Autodesk Fusion 360 part; units mm, degrees
(part 7 of 7)
  spline S1999 degree 3 poles (64.4203, 41.5434) (64.0986, 41.5432) (63.8013, 41.7148) (63.6405, 41.9935) knots 0 0 0 0 1 1 1 1
  spline S2000 degree 3 poles (60.9466, 43.3939) (61.0983, 43.3207) (61.2414, 43.2308) (61.373, 43.1257) knots 0 0 0 0 1 1 1 1
  spline S2001 degree 3 poles (61.9187, 40.2416) (61.7213, 39.8998) (61.4373, 39.6159) (61.0955, 39.4184) knots 0 0 0 0 1 1 1 1
  spline S2002 degree 3 poles (59.9705, 43.6166) (60.1388, 43.6166) (60.3066, 43.5977) (60.4707, 43.5603) knots 0 0 0 0 1 1 1 1
  line L833 (55.8472, 45.7565) -> (55.8472, 45.7565)
  spline S2003 degree 3 poles (59.9705, 39.1166) (59.5755, 39.1167) (59.1875, 39.2208) (58.8455, 39.4184) knots 0 0 0 0 1 1 1 1
  spline S2004 degree 3 poles (63.6405, 42.8937) (63.8013, 43.1723) (64.0986, 43.3439) (64.4203, 43.3438) knots 0 0 0 0 1 1 1 1
  spline S2005 degree 3 poles (61.0955, 39.4184) (60.7535, 39.2208) (60.3655, 39.1167) (59.9705, 39.1166) knots 0 0 0 0 1 1 1 1
  spline S2006 degree 3 poles (50.3545, 46.2686) (49.8082, 46.2688) (49.2842, 46.0518) (48.8978, 45.6656) knots 0 0 0 0 1 1 1 1
  spline S2007 degree 3 poles (42.1917, 76.9836) (42.4279, 76.7471) (42.7484, 76.6142) (43.0826, 76.6141) knots 0 0 0 0 1 1 1 1
  spline S2008 degree 3 poles (58.0218, 40.2416) (57.8243, 40.5837) (57.7204, 40.9717) (57.7205, 41.3666) knots 0 0 0 0 1 1 1 1
  spline S2009 degree 3 poles (58.8455, 43.3153) (59.1875, 43.5128) (59.5755, 43.6167) (59.9705, 43.6166) knots 0 0 0 0 1 1 1 1
  spline S2010 degree 3 poles (58.0218, 42.4916) (58.2193, 42.8337) (58.5034, 43.1178) (58.8455, 43.3153) knots 0 0 0 0 1 1 1 1
  line L834 (59.9705, 43.6166) -> (59.9705, 43.6166)
  spline S2011 degree 3 poles (61.9972, 42.3433) (62.0704, 42.1914) (62.1262, 42.0317) (62.1636, 41.8674) knots 0 0 0 0 1 1 1 1
  line L835 (55.8472, 45.7565) -> (55.8472, 45.7565)
  spline S2012 degree 3 poles (83.1654, 44.538) (83.291, 44.4972) (83.4095, 44.4368) (83.5163, 44.3592) knots 0 0 0 0 1 1 1 1
  spline S2013 degree 3 poles (54.9563, 45.3876) (55.1926, 45.6238) (55.5131, 45.7565) (55.8472, 45.7565) knots 0 0 0 0 1 1 1 1
  line L836 (64.4203, 43.3438) -> (64.4203, 43.3438)
  spline S2014 degree 3 poles (61.373, 43.1257) (61.5048, 43.0207) (61.6244, 42.9013) (61.7295, 42.7696) knots 0 0 0 0 1 1 1 1
  spline S2015 degree 3 poles (60.4707, 43.5603) (60.6351, 43.5228) (60.7947, 43.467) (60.9466, 43.3939) knots 0 0 0 0 1 1 1 1
  spline S2016 degree 3 poles (14.7696, 50.8405) (14.7523, 50.8869) (14.7334, 50.9328) (14.7128, 50.9779) knots 0 0 0 0 1 1 1 1
  spline S2017 degree 3 poles (56.7381, 43.6058) (56.5018, 43.3695) (56.1814, 43.2368) (55.8472, 43.2368) knots 0 0 0 0 1 1 1 1
  spline S2018 degree 3 poles (61.7295, 42.7696) (61.8344, 42.638) (61.9242, 42.495) (61.9972, 42.3433) knots 0 0 0 0 1 1 1 1
  spline S2019 degree 3 poles (55.8472, 43.2368) (55.5131, 43.2368) (55.1926, 43.3695) (54.9563, 43.6058) knots 0 0 0 0 1 1 1 1
  spline S2020 degree 3 poles (58.8455, 39.4184) (58.5034, 39.6158) (58.2193, 39.8997) (58.0218, 40.2416) knots 0 0 0 0 1 1 1 1
  spline S2021 degree 3 poles (57.7205, 41.3666) (57.7204, 41.7616) (57.8243, 42.1496) (58.0218, 42.4916) knots 0 0 0 0 1 1 1 1
  spline S2022 degree 3 poles (83.5163, 44.3592) (83.6234, 44.2814) (83.7176, 44.1872) (83.7954, 44.0802) knots 0 0 0 0 1 1 1 1
  spline S2023 degree 3 poles (42.1917, 78.7654) (41.9555, 78.5291) (41.8227, 78.2086) (41.8228, 77.8745) knots 0 0 0 0 1 1 1 1
  spline S2024 degree 3 poles (57.1071, 44.4967) (57.1071, 44.1625) (56.9744, 43.8421) (56.7381, 43.6058) knots 0 0 0 0 1 1 1 1
  spline S2025 degree 3 poles (54.9563, 45.3876) (54.7199, 45.1514) (54.587, 44.8309) (54.5868, 44.4967) knots 0 0 0 0 1 1 1 1
  spline S2026 degree 3 poles (57.0456, 44.8858) (57.0046, 45.0116) (56.9441, 45.1302) (56.8663, 45.2372) knots 0 0 0 0 1 1 1 1
  spline S2027 degree 3 poles (70.6081, 44.2538) (70.7821, 44.3003) (70.9492, 44.3695) (71.1052, 44.4595) knots 0 0 0 0 1 1 1 1
  spline S2028 degree 3 poles (54.9563, 43.6058) (55.1926, 43.3695) (55.5131, 43.2368) (55.8472, 43.2368) knots 0 0 0 0 1 1 1 1
  line L837 (72.069, 46.7436) -> (71.5853, 46.7436)
  spline S2029 degree 3 poles (71.5093, 39.8938) (71.3486, 39.6154) (71.0515, 39.4438) (70.73, 39.4437) knots 0 0 0 0 1 1 1 1
  line L838 (71.5853, 46.7436) -> (71.5853, 47.6303)
  spline S2030 degree 3 poles (68.6407, 39.8938) (68.4801, 40.1722) (68.4801, 40.5151) (68.6407, 40.7935) knots 0 0 0 0 1 1 1 1
  spline S2031 degree 3 poles (64.4203, 43.3438) (64.0986, 43.3439) (63.8013, 43.1723) (63.6405, 42.8937) knots 0 0 0 0 1 1 1 1
  line L839 (69.42, 41.2436) -> (69.42, 41.2436)
  spline S2032 degree 3 poles (71.1052, 48.0277) (70.9492, 48.1177) (70.7821, 48.1869) (70.6081, 48.2334) knots 0 0 0 0 1 1 1 1
  spline S2033 degree 3 poles (71.5315, 44.7871) (71.6589, 44.9143) (71.769, 45.0576) (71.8592, 45.2134) knots 0 0 0 0 1 1 1 1
  spline S2034 degree 3 poles (63.6839, 45.3524) (63.9202, 45.1162) (64.2407, 44.9834) (64.5748, 44.9835) knots 0 0 0 0 1 1 1 1
  spline S2035 degree 3 poles (71.8592, 45.2134) (71.9492, 45.3694) (72.0183, 45.5366) (72.0648, 45.7105) knots 0 0 0 0 1 1 1 1
  spline S2036 degree 3 poles (65.5944, 46.9844) (65.5168, 47.0912) (65.4228, 47.1852) (65.3159, 47.2629) knots 0 0 0 0 1 1 1 1
  spline S2037 degree 3 poles (57.1071, 44.4967) (57.1071, 44.6288) (57.0864, 44.7601) (57.0456, 44.8858) knots 0 0 0 0 1 1 1 1
  spline S2038 degree 3 poles (70.0753, 44.1835) (70.2552, 44.1836) (70.4343, 44.2072) (70.6081, 44.2538) knots 0 0 0 0 1 1 1 1
  spline S2039 degree 3 poles (56.8663, 45.2372) (56.7886, 45.3441) (56.6946, 45.4381) (56.5877, 45.5157) knots 0 0 0 0 1 1 1 1
  spline S2040 degree 3 poles (64.5748, 44.9835) (64.9092, 44.9833) (65.2298, 45.116) (65.4663, 45.3524) knots 0 0 0 0 1 1 1 1
  spline S2041 degree 3 poles (81.5159, 43.3396) (81.5159, 43.6738) (81.6486, 43.9942) (81.8849, 44.2305) knots 0 0 0 0 1 1 1 1
  spline S2042 degree 3 poles (72.0648, 45.7105) (72.1115, 45.8845) (72.1351, 46.0638) (72.1351, 46.2438) knots 0 0 0 0 1 1 1 1
  spline S2043 degree 3 poles (72.1351, 46.2438) (72.1336, 46.4125) (72.1114, 46.5803) (72.069, 46.7436) knots 0 0 0 0 1 1 1 1
  spline S2044 degree 3 poles (63.6839, 47.1347) (63.4477, 46.8984) (63.315, 46.578) (63.315, 46.2438) knots 0 0 0 0 1 1 1 1
  spline S2045 degree 3 poles (65.4663, 45.3524) (65.7026, 45.5888) (65.8354, 45.9095) (65.8352, 46.2438) knots 0 0 0 0 1 1 1 1
  spline S2046 degree 3 poles (71.5853, 47.6303) (71.5679, 47.654) (71.5499, 47.6772) (71.5315, 47.7001) knots 0 0 0 0 1 1 1 1
  spline S2047 degree 3 poles (84.0357, 43.3396) (84.0357, 43.0055) (83.903, 42.685) (83.6667, 42.4487) knots 0 0 0 0 1 1 1 1
  spline S2048 degree 3 poles (83.6667, 42.4487) (83.4304, 42.2125) (83.1099, 42.0798) (82.7758, 42.0798) knots 0 0 0 0 1 1 1 1
  spline S2049 degree 3 poles (81.8849, 42.4487) (81.6486, 42.685) (81.5159, 43.0055) (81.5159, 43.3396) knots 0 0 0 0 1 1 1 1
  spline S2050 degree 3 poles (56.7381, 43.6058) (56.9744, 43.8421) (57.1071, 44.1625) (57.1071, 44.4967) knots 0 0 0 0 1 1 1 1
  spline S2051 degree 3 poles (63.6405, 42.8937) (63.4797, 42.6151) (63.4797, 42.272) (63.6405, 41.9935) knots 0 0 0 0 1 1 1 1
  spline S2052 degree 3 poles (55.8472, 45.7565) (55.5131, 45.7565) (55.1926, 45.6238) (54.9563, 45.3876) knots 0 0 0 0 1 1 1 1
  spline S2053 degree 3 poles (56.5877, 45.5157) (56.4808, 45.5936) (56.3622, 45.6541) (56.2363, 45.695) knots 0 0 0 0 1 1 1 1
  spline S2054 degree 3 poles (55.8472, 43.2368) (56.1814, 43.2368) (56.5018, 43.3695) (56.7381, 43.6058) knots 0 0 0 0 1 1 1 1
  line L840 (70.73, 39.4437) -> (69.42, 39.4437)
  spline S2055 degree 3 poles (71.5315, 47.7001) (71.4043, 47.8274) (71.261, 47.9376) (71.1052, 48.0277) knots 0 0 0 0 1 1 1 1
  spline S2056 degree 3 poles (68.6407, 40.7935) (68.8015, 41.072) (69.0985, 41.2436) (69.42, 41.2436) knots 0 0 0 0 1 1 1 1
  spline S2057 degree 3 poles (68.6185, 44.7871) (69.0048, 44.4006) (69.5289, 44.1835) (70.0753, 44.1835) knots 0 0 0 0 1 1 1 1
  spline S2058 degree 3 poles (63.6405, 41.9935) (63.8013, 41.7148) (64.0986, 41.5432) (64.4203, 41.5434) knots 0 0 0 0 1 1 1 1
  line L841 (64.4203, 41.5434) -> (65.7303, 41.5434)
  spline S2059 degree 3 poles (66.5096, 41.9935) (66.6705, 42.272) (66.6705, 42.6151) (66.5096, 42.8937) knots 0 0 0 0 1 1 1 1
  spline S2060 degree 3 poles (69.42, 39.4437) (69.0985, 39.4438) (68.8015, 39.6154) (68.6407, 39.8938) knots 0 0 0 0 1 1 1 1
  spline S2061 degree 3 poles (70.0753, 48.3037) (69.5289, 48.3036) (69.0048, 48.0865) (68.6185, 47.7001) knots 0 0 0 0 1 1 1 1
  spline S2062 degree 3 poles (68.0149, 46.2438) (68.015, 45.6974) (68.2321, 45.1734) (68.6185, 44.7871) knots 0 0 0 0 1 1 1 1
  line L842 (64.5748, 47.5037) -> (64.5748, 47.5037)
  spline S2063 degree 3 poles (66.5096, 42.8937) (66.3489, 43.1721) (66.0518, 43.3437) (65.7303, 43.3438) knots 0 0 0 0 1 1 1 1
  line L843 (65.7303, 43.3438) -> (64.4203, 43.3438)
  spline S2064 degree 3 poles (64.5748, 47.5037) (64.2407, 47.5037) (63.9202, 47.371) (63.6839, 47.1347) knots 0 0 0 0 1 1 1 1
  spline S2065 degree 3 poles (54.5868, 44.4967) (54.587, 44.1624) (54.7199, 43.842) (54.9563, 43.6058) knots 0 0 0 0 1 1 1 1
  spline S2066 degree 3 poles (126.6656, 70.8227) (126.2016, 70.8226) (125.7566, 70.6382) (125.4285, 70.3101) knots 0 0 0 0 1 1 1 1
  spline S2067 degree 3 poles (125.4285, 70.3101) (125.1003, 69.982) (124.9159, 69.537) (124.9159, 69.0729) knots 0 0 0 0 1 1 1 1
  spline S2068 degree 3 poles (64.9645, 47.4417) (64.8387, 47.4827) (64.7072, 47.5036) (64.5748, 47.5037) knots 0 0 0 0 1 1 1 1
  spline S2069 degree 3 poles (126.6656, 67.3227) (127.1298, 67.3226) (127.575, 67.507) (127.9033, 67.8353) knots 0 0 0 0 1 1 1 1
  spline S2070 degree 3 poles (65.7303, 41.5434) (66.0518, 41.5434) (66.3489, 41.715) (66.5096, 41.9935) knots 0 0 0 0 1 1 1 1
  spline S2071 degree 3 poles (82.7758, 42.0798) (82.4417, 42.0798) (82.1212, 42.2125) (81.8849, 42.4487) knots 0 0 0 0 1 1 1 1
  spline S2072 degree 3 poles (83.9742, 43.7287) (84.0149, 43.6031) (84.0357, 43.4718) (84.0357, 43.3396) knots 0 0 0 0 1 1 1 1
  spline S2073 degree 3 poles (81.8849, 44.2305) (82.1212, 44.4668) (82.4417, 44.5995) (82.7758, 44.5995) knots 0 0 0 0 1 1 1 1
  spline S2074 degree 3 poles (71.1052, 44.4595) (71.261, 44.5496) (71.4043, 44.6597) (71.5315, 44.7871) knots 0 0 0 0 1 1 1 1
  spline S2075 degree 3 poles (68.6185, 47.7001) (68.2322, 47.3139) (68.0151, 46.7901) (68.0149, 46.2438) knots 0 0 0 0 1 1 1 1
  line L844 (82.7758, 44.5995) -> (82.7758, 44.5995)
  spline S2076 degree 3 poles (63.315, 46.2438) (63.3148, 45.9095) (63.4476, 45.5888) (63.6839, 45.3524) knots 0 0 0 0 1 1 1 1
  spline S2077 degree 3 poles (65.8352, 46.2438) (65.8351, 46.376) (65.8142, 46.5073) (65.7732, 46.633) knots 0 0 0 0 1 1 1 1
  spline S2078 degree 3 poles (65.3159, 47.2629) (65.2089, 47.3406) (65.0903, 47.4009) (64.9645, 47.4417) knots 0 0 0 0 1 1 1 1
  spline S2079 degree 3 poles (65.7732, 46.633) (65.7324, 46.7588) (65.6721, 46.8773) (65.5944, 46.9844) knots 0 0 0 0 1 1 1 1
  spline S2080 degree 3 poles (70.6081, 48.2334) (70.4343, 48.28) (70.2552, 48.3036) (70.0753, 48.3037) knots 0 0 0 0 1 1 1 1
  line L845 (83.1458, 68.537) -> (85.7053, 68.4921)
  spline S2081 degree 3 poles (52.0676, 69.0326) (52.0731, 68.8996) (52.132, 68.7744) (52.2309, 68.6854) knots 0 0 0 0 1 1 1 1
  spline S2082 degree 3 poles (124.9159, 69.0729) (124.9158, 68.6087) (125.1002, 68.1635) (125.4285, 67.8353) knots 0 0 0 0 1 1 1 1
  spline S2083 degree 3 poles (127.1188, 70.7633) (126.971, 70.8028) (126.8186, 70.8228) (126.6656, 70.8227) knots 0 0 0 0 1 1 1 1
  spline S2084 degree 3 poles (110.3875, 62.1504) (110.4782, 62.0529) (110.6043, 61.9961) (110.7374, 61.9927) knots 0 0 0 0 1 1 1 1
  line L846 (115.0007, 55.1399) -> (108.505, 55.3668)
  spline S2085 degree 3 poles (91.7158, 67.8875) (91.712, 67.7545) (91.762, 67.6256) (91.8543, 67.5299) knots 0 0 0 0 1 1 1 1
  line L847 (86.095, 63.8846) -> (83.0652, 63.9378)
  spline S2086 degree 3 poles (90.1066, 61.6646) (90.0648, 62.0236) (89.8898, 62.3539) (89.6162, 62.5901) knots 0 0 0 0 1 1 1 1
  line L848 (110.2904, 63.5094) -> (110.2553, 62.51)
  spline S2087 degree 3 poles (128.3559, 69.5256) (128.3164, 69.6734) (128.2577, 69.8153) (128.1813, 69.9478) knots 0 0 0 0 1 1 1 1
  line L849 (59.9596, 63.1875) -> (57.3882, 63.0526)
  spline S2088 degree 3 poles (91.8543, 67.5299) (91.9467, 67.4341) (92.0737, 67.3795) (92.2067, 67.3785) knots 0 0 0 0 1 1 1 1
  spline S2089 degree 3 poles (128.4159, 69.0729) (128.4158, 69.2258) (128.3956, 69.378) (128.3559, 69.5256) knots 0 0 0 0 1 1 1 1
  line L850 (99.2606, 66.1052) -> (99.1805, 61.506)
  line L851 (104.5657, 58.6064) -> (101.5374, 58.7118)
  spline S2090 degree 3 poles (125.4285, 67.8353) (125.7566, 67.5071) (126.2016, 67.3227) (126.6656, 67.3227) knots 0 0 0 0 1 1 1 1
  line L852 (109.8077, 64.0267) -> (110.2904, 63.5094)
  line L853 (104.8111, 64.2014) -> (109.8077, 64.0267)
  line L854 (115.2348, 61.8362) -> (115.1945, 60.6869)
  line L855 (117.768, 60.597) -> (117.6078, 55.9998)
  spline S2091 degree 3 poles (128.1813, 69.9478) (128.1048, 70.0802) (128.0114, 70.202) (127.9033, 70.3101) knots 0 0 0 0 1 1 1 1
  line L856 (107.0823, 57.6178) -> (105.4834, 57.6736)
  line L857 (104.2732, 63.6996) -> (104.8111, 64.2014)
  line L858 (101.6982, 63.3095) -> (104.2561, 63.2201)
  line L859 (99.1805, 61.506) -> (96.606, 61.5509)
  line L860 (96.5894, 60.6011) -> (90.0901, 60.7148)
  line L861 (96.6861, 66.1501) -> (99.2606, 66.1052)
  spline S2092 degree 3 poles (89.6162, 62.5901) (89.3425, 62.8265) (88.9901, 62.9515) (88.6287, 62.9405) knots 0 0 0 0 1 1 1 1
  line L862 (90.0901, 60.7148) -> (90.1066, 61.6646)
  line L863 (51.4899, 70.5044) -> (52.0154, 70.031)
  spline S2093 degree 3 poles (108.0637, 57.2504) (107.7941, 57.4915) (107.4439, 57.6226) (107.0823, 57.6178) knots 0 0 0 0 1 1 1 1
  spline S2094 degree 3 poles (127.9033, 70.3101) (127.795, 70.4184) (127.6731, 70.512) (127.5405, 70.5886) knots 0 0 0 0 1 1 1 1
  line L864 (88.6287, 62.9405) -> (87.0293, 62.9684)
  line L865 (52.0154, 70.031) -> (52.0676, 69.0326)
  line L866 (115.1945, 60.6869) -> (117.768, 60.597)
  spline S2095 degree 3 poles (50.8971, 62.7126) (50.8304, 63.068) (50.6327, 63.3853) (50.3432, 63.602) knots 0 0 0 0 1 1 1 1
  line L867 (117.6078, 55.9998) -> (115.0343, 56.0892)
  line L868 (85.7136, 68.9722) -> (86.2428, 69.4832)
  line L869 (104.2561, 63.2201) -> (104.2732, 63.6996)
  line L870 (59.7188, 67.781) -> (59.9596, 63.1875)
  spline S2096 degree 3 poles (110.2553, 62.51) (110.2493, 62.3772) (110.2969, 62.2476) (110.3875, 62.1504) knots 0 0 0 0 1 1 1 1
  line L871 (96.7062, 67.2999) -> (96.6861, 66.1501)
  line L872 (83.0652, 63.9378) -> (83.1458, 68.537)
  line L873 (108.505, 55.3668) -> (108.538, 56.3161)
  line L874 (86.2428, 69.4832) -> (91.2419, 69.3959)
  line L875 (57.0869, 68.7949) -> (57.1474, 67.6461)
  line L876 (85.7053, 68.4921) -> (85.7136, 68.9722)
  spline S2097 degree 3 poles (52.2309, 68.6854) (52.3298, 68.5963) (52.4604, 68.5509) (52.5932, 68.5593) knots 0 0 0 0 1 1 1 1
  line L877 (52.5932, 68.5593) -> (57.0869, 68.7949)
  line L878 (57.3882, 63.0526) -> (57.4378, 62.1039)
  spline S2098 degree 3 poles (108.538, 56.3161) (108.5025, 56.6759) (108.3332, 57.0094) (108.0637, 57.2504) knots 0 0 0 0 1 1 1 1
  line L879 (126.6656, 70.8227) -> (126.6656, 70.8227)
  line L880 (105.4834, 57.6736) -> (104.5657, 58.6064)
  line L881 (91.2419, 69.3959) -> (91.7334, 68.8869)
  spline S2099 degree 3 poles (127.9033, 67.8353) (128.2315, 68.1635) (128.4159, 68.6087) (128.4159, 69.0729) knots 0 0 0 0 1 1 1 1
  spline S2100 degree 3 poles (127.5405, 70.5886) (127.4082, 70.665) (127.2664, 70.7237) (127.1188, 70.7633) knots 0 0 0 0 1 1 1 1
  line L882 (115.0343, 56.0892) -> (115.0007, 55.1399)
  line L883 (91.7334, 68.8869) -> (91.7158, 67.8875)
  line L884 (96.606, 61.5509) -> (96.5894, 60.6011)
  line L885 (92.2067, 67.3785) -> (96.7062, 67.2999)
  line L886 (101.5374, 58.7118) -> (101.6982, 63.3095)
  line L887 (110.7374, 61.9927) -> (115.2348, 61.8362)
  line L888 (87.0293, 62.9684) -> (86.095, 63.8846)
  spline S2101 degree 3 poles (128.1813, 69.9478) (128.2577, 69.8153) (128.3164, 69.6734) (128.3559, 69.5256) knots 0 0 0 0 1 1 1 1
  line L889 (47.7356, 63.7983) -> (46.7398, 64.6474)
  spline S2102 degree 3 poles (103.8898, 68.6854) (104.0402, 68.4018) (104.0282, 68.0596) (103.8582, 67.7872) knots 0 0 0 0 1 1 1 1
  line L890 (49.3334, 63.882) -> (47.7356, 63.7983)
  line L891 (103.0655, 67.364) -> (101.756, 67.41)
  spline S2103 degree 3 poles (89.6121, 37.7689) (89.7676, 37.488) (89.7616, 37.1456) (89.5966, 36.8703) knots 0 0 0 0 1 1 1 1
  line L892 (46.7398, 64.6474) -> (43.7141, 64.4892)
  line L893 (46.0297, 69.2166) -> (46.0049, 69.6962)
  spline S2104 degree 3 poles (127.5405, 70.5886) (127.6731, 70.512) (127.795, 70.4184) (127.9033, 70.3101) knots 0 0 0 0 1 1 1 1
  spline S2105 degree 3 poles (101.756, 67.41) (101.4352, 67.4218) (101.145, 67.6035) (100.9943, 67.887) knots 0 0 0 0 1 1 1 1
  line L894 (88.8426, 38.233) -> (87.5331, 38.2557)
  line L895 (88.8111, 36.4331) -> (87.5016, 36.4563)
  line L896 (57.1474, 67.6461) -> (59.7188, 67.781)
  spline S2106 degree 3 poles (88.8111, 36.4331) (89.1322, 36.4282) (89.4315, 36.5948) (89.5966, 36.8703) knots 0 0 0 0 1 1 1 1
  spline S2107 degree 3 poles (89.6121, 37.7689) (89.4567, 38.0497) (89.1635, 38.2265) (88.8426, 38.233) knots 0 0 0 0 1 1 1 1
  spline S2108 degree 3 poles (88.8426, 38.233) (89.1635, 38.2265) (89.4567, 38.0497) (89.6121, 37.7689) knots 0 0 0 0 1 1 1 1
  spline S2109 degree 3 poles (86.7321, 36.9204) (86.5767, 37.2013) (86.5826, 37.5437) (86.7476, 37.819) knots 0 0 0 0 1 1 1 1
  line L897 (43.7141, 64.4892) -> (43.4733, 69.0828)
  line L898 (87.5016, 36.4563) -> (88.8111, 36.4331)
  spline S2110 degree 3 poles (86.7476, 37.819) (86.9129, 38.0943) (87.2122, 38.2606) (87.5331, 38.2557) knots 0 0 0 0 1 1 1 1
  line L899 (43.4733, 69.0828) -> (46.0297, 69.2166)
  spline S2111 degree 3 poles (100.9943, 67.887) (100.8437, 68.1707) (100.8557, 68.5131) (101.0258, 68.7856) knots 0 0 0 0 1 1 1 1
  line L900 (87.5331, 38.2557) -> (87.5331, 38.2557)
  spline S2112 degree 3 poles (81.7852, 40.0055) (81.6201, 39.7303) (81.614, 39.3882) (81.7691, 39.1073) knots 0 0 0 0 1 1 1 1
  spline S2113 degree 3 poles (81.7691, 39.1073) (81.9246, 38.8264) (82.2181, 38.6495) (82.5391, 38.6433) knots 0 0 0 0 1 1 1 1
  line L901 (82.5391, 38.6433) -> (83.8486, 38.62)
  line L902 (82.5701, 40.4426) -> (83.8801, 40.4199)
  spline S2114 degree 3 poles (84.6496, 39.9559) (84.8051, 39.675) (84.7992, 39.3325) (84.6341, 39.0572) knots 0 0 0 0 1 1 1 1
  spline S2115 degree 3 poles (84.6341, 39.0572) (84.469, 38.7818) (84.1697, 38.6152) (83.8486, 38.62) knots 0 0 0 0 1 1 1 1
  spline S2116 degree 3 poles (69.42, 41.2436) (69.0985, 41.2436) (68.8015, 41.072) (68.6407, 40.7935) knots 0 0 0 0 1 1 1 1
  spline S2117 degree 3 poles (87.5016, 36.4563) (87.1807, 36.4627) (86.8875, 36.6396) (86.7321, 36.9204) knots 0 0 0 0 1 1 1 1
  spline S2118 degree 3 poles (50.3432, 63.602) (50.0535, 63.8185) (49.6932, 63.9184) (49.3334, 63.882) knots 0 0 0 0 1 1 1 1
  spline S2119 degree 3 poles (81.7691, 39.1073) (81.614, 39.3882) (81.6201, 39.7303) (81.7852, 40.0055) knots 0 0 0 0 1 1 1 1
  spline S2120 degree 3 poles (89.5966, 36.8703) (89.7616, 37.1456) (89.7676, 37.488) (89.6121, 37.7689) knots 0 0 0 0 1 1 1 1
  line L903 (50.9467, 61.7638) -> (50.8971, 62.7126)
  line L904 (46.0049, 69.6962) -> (46.4969, 70.2424)
  spline S2121 degree 3 poles (127.1188, 70.7633) (127.2664, 70.7237) (127.4082, 70.665) (127.5405, 70.5886) knots 0 0 0 0 1 1 1 1
  line L905 (87.5331, 38.2557) -> (88.8426, 38.233)
  spline S2122 degree 3 poles (84.6341, 39.0572) (84.7992, 39.3325) (84.8051, 39.675) (84.6496, 39.9559) knots 0 0 0 0 1 1 1 1
  spline S2123 degree 3 poles (84.6496, 39.9559) (84.4942, 40.2367) (84.201, 40.4135) (83.8801, 40.4199) knots 0 0 0 0 1 1 1 1
  line L906 (101.8191, 69.2088) -> (103.128, 69.1628)
  spline S2124 degree 3 poles (89.5966, 36.8703) (89.4315, 36.5948) (89.1322, 36.4282) (88.8111, 36.4331) knots 0 0 0 0 1 1 1 1
  spline S2125 degree 3 poles (127.9033, 70.3101) (128.0114, 70.202) (128.1048, 70.0802) (128.1813, 69.9478) knots 0 0 0 0 1 1 1 1
  spline S2126 degree 3 poles (81.7852, 40.0055) (81.9502, 40.2807) (82.2492, 40.4473) (82.5701, 40.4426) knots 0 0 0 0 1 1 1 1
  spline S2127 degree 3 poles (68.6407, 40.7935) (68.4801, 40.5151) (68.4801, 40.1722) (68.6407, 39.8938) knots 0 0 0 0 1 1 1 1
  spline S2128 degree 3 poles (126.6656, 70.8227) (126.8186, 70.8228) (126.971, 70.8028) (127.1188, 70.7633) knots 0 0 0 0 1 1 1 1
  spline S2129 degree 3 poles (101.0258, 68.7856) (101.1958, 69.0581) (101.4981, 69.2194) (101.8191, 69.2088) knots 0 0 0 0 1 1 1 1
  spline S2130 degree 3 poles (68.6407, 39.8938) (68.8015, 39.6154) (69.0985, 39.4438) (69.42, 39.4437) knots 0 0 0 0 1 1 1 1
  line L907 (83.8486, 38.62) -> (82.5391, 38.6433)
  line L908 (69.42, 39.4437) -> (70.73, 39.4437)
  spline S2131 degree 3 poles (70.73, 39.4437) (71.0515, 39.4438) (71.3486, 39.6154) (71.5093, 39.8938) knots 0 0 0 0 1 1 1 1
  spline S2132 degree 3 poles (82.5391, 38.6433) (82.2181, 38.6495) (81.9246, 38.8264) (81.7691, 39.1073) knots 0 0 0 0 1 1 1 1
  spline S2133 degree 3 poles (71.5093, 39.8938) (71.67, 40.1722) (71.67, 40.5151) (71.5093, 40.7935) knots 0 0 0 0 1 1 1 1
  spline S2134 degree 3 poles (83.8801, 40.4199) (84.201, 40.4135) (84.4942, 40.2367) (84.6496, 39.9559) knots 0 0 0 0 1 1 1 1
  line L909 (82.5701, 40.4426) -> (82.5701, 40.4426)
  line L910 (46.4969, 70.2424) -> (51.4899, 70.5044)
  line L911 (57.4378, 62.1039) -> (50.9467, 61.7638)
  spline S2135 degree 3 poles (128.3559, 69.5256) (128.3956, 69.378) (128.4158, 69.2258) (128.4159, 69.0729) knots 0 0 0 0 1 1 1 1
  spline S2136 degree 3 poles (103.128, 69.1628) (103.4489, 69.151) (103.7392, 68.969) (103.8898, 68.6854) knots 0 0 0 0 1 1 1 1
  spline S2137 degree 3 poles (103.8582, 67.7872) (103.6884, 67.5149) (103.3863, 67.3536) (103.0655, 67.364) knots 0 0 0 0 1 1 1 1
  line L912 (101.8191, 69.2088) -> (101.8191, 69.2088)
  spline S2138 degree 3 poles (82.5701, 40.4426) (82.2492, 40.4473) (81.9502, 40.2807) (81.7852, 40.0055) knots 0 0 0 0 1 1 1 1
  spline S2139 degree 3 poles (83.8486, 38.62) (84.1697, 38.6152) (84.469, 38.7818) (84.6341, 39.0572) knots 0 0 0 0 1 1 1 1
  line L913 (83.8801, 40.4199) -> (82.5701, 40.4426)
  line L914 (50.3545, 46.2686) -> (50.3545, 46.2686)
  spline S2140 degree 3 poles (52.3446, 43.6755) (52.2979, 43.5017) (52.2285, 43.3347) (52.1384, 43.1789) knots 0 0 0 0 1 1 1 1
  spline S2141 degree 3 poles (83.6667, 42.4487) (83.903, 42.685) (84.0357, 43.0055) (84.0357, 43.3396) knots 0 0 0 0 1 1 1 1
  spline S2142 degree 3 poles (92.8832, 42.2565) (93.1195, 42.0202) (93.4399, 41.8875) (93.7741, 41.8875) knots 0 0 0 0 1 1 1 1
  spline S2143 degree 3 poles (48.8978, 45.6656) (49.2842, 46.0518) (49.8082, 46.2688) (50.3545, 46.2686) knots 0 0 0 0 1 1 1 1
  spline S2144 degree 3 poles (92.5142, 43.1474) (92.5142, 42.8132) (92.6469, 42.4928) (92.8832, 42.2565) knots 0 0 0 0 1 1 1 1
  line L915 (69.42, 41.2436) -> (70.73, 41.2436)
  spline S2145 degree 3 poles (51.8113, 45.6656) (51.9385, 45.5382) (52.0485, 45.3947) (52.1384, 45.2387) knots 0 0 0 0 1 1 1 1
  spline S2146 degree 3 poles (51.8113, 42.7521) (51.6839, 42.6248) (51.5404, 42.5149) (51.3844, 42.425) knots 0 0 0 0 1 1 1 1
  spline S2147 degree 3 poles (81.8849, 44.2305) (81.6486, 43.9942) (81.5159, 43.6738) (81.5159, 43.3396) knots 0 0 0 0 1 1 1 1
  spline S2148 degree 3 poles (82.7758, 42.0798) (83.1099, 42.0798) (83.4304, 42.2125) (83.6667, 42.4487) knots 0 0 0 0 1 1 1 1
  spline S2149 degree 3 poles (83.7954, 44.0802) (83.7176, 44.1872) (83.6234, 44.2814) (83.5163, 44.3592) knots 0 0 0 0 1 1 1 1
  spline S2150 degree 3 poles (51.3844, 42.425) (51.2286, 42.3348) (51.0617, 42.2655) (50.8878, 42.2188) knots 0 0 0 0 1 1 1 1
  spline S2151 degree 3 poles (93.7741, 41.8875) (94.1082, 41.8875) (94.4287, 42.0202) (94.665, 42.2565) knots 0 0 0 0 1 1 1 1
  spline S2152 degree 3 poles (71.5093, 40.7935) (71.3486, 41.072) (71.0515, 41.2436) (70.73, 41.2436) knots 0 0 0 0 1 1 1 1
  spline S2153 degree 3 poles (84.0357, 43.3396) (84.0357, 43.4718) (84.0149, 43.6031) (83.9742, 43.7287) knots 0 0 0 0 1 1 1 1
  line L916 (82.7758, 44.5995) -> (82.7758, 44.5995)
  spline S2154 degree 3 poles (74.522, 46.7436) (74.4176, 46.5939) (74.3469, 46.4235) (74.3148, 46.2438) knots 0 0 0 0 1 1 1 1
  spline S2155 degree 3 poles (76.4661, 45.3524) (76.7025, 45.5888) (76.8352, 45.9095) (76.8351, 46.2438) knots 0 0 0 0 1 1 1 1
  spline S2156 degree 3 poles (75.5752, 44.9835) (75.9094, 44.9834) (76.2298, 45.1162) (76.4661, 45.3524) knots 0 0 0 0 1 1 1 1
  spline S2157 degree 3 poles (94.9725, 43.537) (94.9584, 43.5678) (94.943, 43.5979) (94.9265, 43.6275) knots 0 0 0 0 1 1 1 1
  spline S2158 degree 3 poles (76.7736, 46.633) (76.7566, 46.6707) (76.7378, 46.7076) (76.7173, 46.7436) knots 0 0 0 0 1 1 1 1
  spline S2159 degree 3 poles (71.5093, 40.7935) (71.67, 40.5151) (71.67, 40.1722) (71.5093, 39.8938) knots 0 0 0 0 1 1 1 1
  spline S2160 degree 3 poles (50.3545, 42.1485) (49.8081, 42.1485) (49.2841, 42.3656) (48.8978, 42.7521) knots 0 0 0 0 1 1 1 1
  spline S2161 degree 3 poles (48.8978, 42.7521) (48.5115, 43.1385) (48.2946, 43.6625) (48.2947, 44.2088) knots 0 0 0 0 1 1 1 1
  spline S2162 degree 3 poles (83.5163, 44.3592) (83.4095, 44.4368) (83.291, 44.4972) (83.1654, 44.538) knots 0 0 0 0 1 1 1 1
  spline S2163 degree 3 poles (82.7758, 44.5995) (82.4417, 44.5995) (82.1212, 44.4668) (81.8849, 44.2305) knots 0 0 0 0 1 1 1 1
  line L917 (64.4203, 43.3438) -> (65.7303, 43.3438)
  spline S2164 degree 3 poles (66.5096, 41.9935) (66.3489, 41.715) (66.0518, 41.5434) (65.7303, 41.5434) knots 0 0 0 0 1 1 1 1
  spline S2165 degree 3 poles (50.8878, 46.1984) (51.0616, 46.1518) (51.2286, 46.0826) (51.3844, 45.9927) knots 0 0 0 0 1 1 1 1
  spline S2166 degree 3 poles (95.0345, 43.1474) (95.0344, 43.2797) (95.0135, 43.4112) (94.9725, 43.537) knots 0 0 0 0 1 1 1 1
  line L918 (76.7173, 46.7436) -> (74.522, 46.7436)
  spline S2167 degree 3 poles (83.9742, 43.7287) (83.9334, 43.8545) (83.873, 43.9731) (83.7954, 44.0802) knots 0 0 0 0 1 1 1 1
  line L919 (65.7303, 41.5434) -> (64.4203, 41.5434)
  spline S2168 degree 3 poles (52.1384, 45.2387) (52.2285, 45.0829) (52.2979, 44.916) (52.3446, 44.7421) knots 0 0 0 0 1 1 1 1
  spline S2169 degree 3 poles (74.6843, 45.3524) (74.9206, 45.1162) (75.2411, 44.9834) (75.5752, 44.9835) knots 0 0 0 0 1 1 1 1
  spline S2170 degree 3 poles (83.1654, 44.538) (83.0396, 44.5788) (82.9081, 44.5996) (82.7758, 44.5995) knots 0 0 0 0 1 1 1 1
  spline S2171 degree 3 poles (52.3446, 44.7421) (52.3911, 44.5682) (52.4145, 44.3889) (52.4144, 44.2088) knots 0 0 0 0 1 1 1 1
  spline S2172 degree 3 poles (12.7801, 48.2473) (12.2337, 48.2472) (11.7097, 48.4642) (11.3233, 48.8504) knots 0 0 0 0 1 1 1 1
  spline S2173 degree 3 poles (13.3134, 48.3171) (13.1394, 48.2706) (12.9601, 48.2472) (12.7801, 48.2473) knots 0 0 0 0 1 1 1 1
  spline S2174 degree 3 poles (11.3233, 48.8504) (10.9371, 49.2368) (10.7202, 49.7608) (10.7203, 50.3072) knots 0 0 0 0 1 1 1 1
  spline S2175 degree 3 poles (92.7287, 43.6662) (92.6191, 43.5116) (92.5458, 43.3343) (92.5142, 43.1474) knots 0 0 0 0 1 1 1 1
  spline S2176 degree 3 poles (11.3233, 51.7639) (11.7097, 52.1502) (12.2337, 52.3671) (12.7801, 52.367) knots 0 0 0 0 1 1 1 1
  spline S2177 degree 3 poles (10.7203, 50.3072) (10.7202, 50.8535) (10.9371, 51.3775) (11.3233, 51.7639) knots 0 0 0 0 1 1 1 1
  spline S2178 degree 3 poles (74.3148, 46.2438) (74.3148, 45.9094) (74.4477, 45.5888) (74.6843, 45.3524) knots 0 0 0 0 1 1 1 1
  spline S2179 degree 3 poles (13.3134, 52.2967) (13.4872, 52.2501) (13.6542, 52.181) (13.81, 52.091) knots 0 0 0 0 1 1 1 1
  spline S2180 degree 3 poles (13.81, 52.091) (13.9373, 52.0138) (14.0558, 51.923) (14.1635, 51.8202) knots 0 0 0 0 1 1 1 1
  spline S2181 degree 3 poles (48.2947, 44.2088) (48.2946, 44.7552) (48.5115, 45.2792) (48.8978, 45.6656) knots 0 0 0 0 1 1 1 1
  spline S2182 degree 3 poles (81.8849, 42.4487) (82.1212, 42.2125) (82.4417, 42.0798) (82.7758, 42.0798) knots 0 0 0 0 1 1 1 1
  line L920 (14.1635, 51.8202) -> (14.1578, 51.8833)
  spline S2183 degree 3 poles (12.7801, 52.367) (12.9602, 52.367) (13.1395, 52.3433) (13.3134, 52.2967) knots 0 0 0 0 1 1 1 1
  spline S2184 degree 3 poles (65.7303, 43.3438) (66.0518, 43.3437) (66.3489, 43.1721) (66.5096, 42.8937) knots 0 0 0 0 1 1 1 1
  spline S2185 degree 3 poles (81.5159, 43.3396) (81.5159, 43.0055) (81.6486, 42.685) (81.8849, 42.4487) knots 0 0 0 0 1 1 1 1
  spline S2186 degree 3 poles (70.73, 41.2436) (71.0515, 41.2436) (71.3486, 41.072) (71.5093, 40.7935) knots 0 0 0 0 1 1 1 1
  spline S2187 degree 3 poles (50.3545, 46.2686) (50.5346, 46.2686) (50.7139, 46.245) (50.8878, 46.1984) knots 0 0 0 0 1 1 1 1
  line L921 (70.73, 41.2436) -> (69.42, 41.2436)
  spline S2188 degree 3 poles (94.665, 42.2565) (94.9014, 42.4927) (95.0343, 42.8132) (95.0345, 43.1474) knots 0 0 0 0 1 1 1 1
  spline S2189 degree 3 poles (76.8351, 46.2438) (76.8351, 46.376) (76.8144, 46.5073) (76.7736, 46.633) knots 0 0 0 0 1 1 1 1
  spline S2190 degree 3 poles (66.5096, 42.8937) (66.6705, 42.6151) (66.6705, 42.272) (66.5096, 41.9935) knots 0 0 0 0 1 1 1 1
  line L922 (94.9265, 43.6275) -> (92.7287, 43.6662)
  spline S2191 degree 3 poles (51.3844, 45.9927) (51.5404, 45.9028) (51.6839, 45.7928) (51.8113, 45.6656) knots 0 0 0 0 1 1 1 1
  spline S2192 degree 3 poles (52.1384, 43.1789) (52.0485, 43.023) (51.9385, 42.8794) (51.8113, 42.7521) knots 0 0 0 0 1 1 1 1
  spline S2193 degree 3 poles (50.8878, 42.2188) (50.7139, 42.1721) (50.5346, 42.1485) (50.3545, 42.1485) knots 0 0 0 0 1 1 1 1
  spline S2194 degree 3 poles (52.4144, 44.2088) (52.4145, 44.0288) (52.3911, 43.8495) (52.3446, 43.6755) knots 0 0 0 0 1 1 1 1
  spline S2195 degree 3 poles (14.1578, 51.8833) (14.0786, 52.236) (13.8701, 52.5461) (13.5733, 52.7525) knots 0 0 0 0 1 1 1 1
  line L923 (6.9174, 53.4077) -> (6.5164, 57.9904)
  line L924 (12.5548, 52.998) -> (10.9606, 52.8584)
  line L925 (9.0666, 58.2137) -> (9.0248, 58.6917)
  line L926 (9.0248, 58.6917) -> (9.4976, 59.2549)
  line L927 (9.4976, 59.2549) -> (14.4787, 59.6911)
  line L928 (9.9358, 53.6718) -> (6.9174, 53.4077)
  line L929 (10.9606, 52.8584) -> (9.9358, 53.6718)
  line L930 (6.5164, 57.9904) -> (9.0666, 58.2137)
  spline S2196 degree 3 poles (8.4992, 50.2172) (8.5402, 50.0914) (8.5611, 49.9599) (8.5612, 49.8276) knots 0 0 0 0 1 1 1 1
  spline S2197 degree 3 poles (8.3204, 49.0871) (8.2426, 48.9802) (8.1484, 48.8862) (8.0414, 48.8085) knots 0 0 0 0 1 1 1 1
  spline S2198 degree 3 poles (13.5733, 52.7525) (13.2765, 52.959) (12.9131, 53.0466) (12.5548, 52.998) knots 0 0 0 0 1 1 1 1
  spline S2199 degree 3 poles (8.4992, 49.4385) (8.4584, 49.3127) (8.3981, 49.1941) (8.3204, 49.0871) knots 0 0 0 0 1 1 1 1
  spline S2200 degree 3 poles (8.0414, 48.8085) (7.9345, 48.7307) (7.8161, 48.6702) (7.6905, 48.6292) knots 0 0 0 0 1 1 1 1
  spline S2201 degree 3 poles (8.0414, 50.8472) (8.1485, 50.7694) (8.2426, 50.6752) (8.3204, 50.5681) knots 0 0 0 0 1 1 1 1
  spline S2202 degree 3 poles (6.4099, 48.9367) (6.1737, 49.173) (6.041, 49.4935) (6.041, 49.8276) knots 0 0 0 0 1 1 1 1
  spline S2203 degree 3 poles (8.3204, 50.5681) (8.398, 50.4613) (8.4584, 50.3429) (8.4992, 50.2172) knots 0 0 0 0 1 1 1 1
  spline S2204 degree 3 poles (6.041, 49.8276) (6.041, 50.1617) (6.1737, 50.4822) (6.4099, 50.7185) knots 0 0 0 0 1 1 1 1
  spline S2205 degree 3 poles (7.3008, 48.5677) (6.9667, 48.5677) (6.6462, 48.7004) (6.4099, 48.9367) knots 0 0 0 0 1 1 1 1
  line L931 (7.3008, 51.088) -> (7.3008, 51.088)
  spline S2206 degree 3 poles (7.6905, 48.6292) (7.5646, 48.5884) (7.4331, 48.5676) (7.3008, 48.5677) knots 0 0 0 0 1 1 1 1
  spline S2207 degree 3 poles (8.7829, 47.0428) (9.0761, 47.0423) (9.3507, 46.899) (9.5188, 46.6588) knots 0 0 0 0 1 1 1 1
  spline S2208 degree 3 poles (7.3008, 51.088) (7.4332, 51.0879) (7.5647, 51.067) (7.6905, 51.026) knots 0 0 0 0 1 1 1 1
  spline S2209 degree 3 poles (8.5612, 49.8276) (8.5611, 49.6954) (8.5402, 49.5641) (8.4992, 49.4385) knots 0 0 0 0 1 1 1 1
  spline S2210 degree 3 poles (7.6905, 51.026) (7.8161, 50.9851) (7.9345, 50.9248) (8.0414, 50.8472) knots 0 0 0 0 1 1 1 1
  spline S2211 degree 3 poles (6.4099, 50.7185) (6.6462, 50.9549) (6.9666, 51.0879) (7.3008, 51.088) knots 0 0 0 0 1 1 1 1
  line L932 (8.8615, 45.2465) -> (7.5561, 45.1323)
  spline S2212 degree 3 poles (9.5188, 46.6588) (9.7031, 46.3956) (9.733, 46.054) (9.5973, 45.7627) knots 0 0 0 0 1 1 1 1
  spline S2213 degree 3 poles (14.1423, 78.4098) (14.1026, 78.5576) (14.0437, 78.6996) (13.9671, 78.832) knots 0 0 0 0 1 1 1 1
  spline S2214 degree 3 poles (10.7017, 77.9566) (10.7018, 77.4926) (10.8862, 77.0476) (11.2143, 76.7195) knots 0 0 0 0 1 1 1 1
  spline S2215 degree 3 poles (11.2143, 76.7195) (11.5425, 76.3912) (11.9877, 76.2068) (12.4519, 76.2069) knots 0 0 0 0 1 1 1 1
  spline S2216 degree 3 poles (107.842, 36.4734) (107.9692, 36.6008) (108.0792, 36.7443) (108.1691, 36.9002) knots 0 0 0 0 1 1 1 1
  spline S2217 degree 3 poles (13.9671, 78.832) (13.8906, 78.9644) (13.7972, 79.0862) (13.6891, 79.1943) knots 0 0 0 0 1 1 1 1
  spline S2218 degree 3 poles (108.445, 37.9301) (108.4413, 38.0752) (108.4222, 38.2195) (108.3882, 38.3606) knots 0 0 0 0 1 1 1 1
  line L933 (108.3882, 38.3606) -> (107.9117, 38.3771)
  spline S2219 degree 3 poles (11.2143, 79.1943) (10.886, 78.866) (10.7016, 78.4208) (10.7017, 77.9566) knots 0 0 0 0 1 1 1 1
  spline S2220 degree 3 poles (12.4519, 79.7069) (11.9877, 79.7069) (11.5425, 79.5225) (11.2143, 79.1943) knots 0 0 0 0 1 1 1 1
  line L934 (107.9117, 38.3771) -> (107.9422, 39.2562)
  spline S2221 degree 3 poles (14.2017, 77.9566) (14.2018, 78.1096) (14.1818, 78.262) (14.1423, 78.4098) knots 0 0 0 0 1 1 1 1
  spline S2222 degree 3 poles (13.6891, 76.7195) (14.0172, 77.0476) (14.2016, 77.4926) (14.2017, 77.9566) knots 0 0 0 0 1 1 1 1
  spline S2223 degree 3 poles (108.1691, 36.9002) (108.259, 37.0561) (108.3282, 37.223) (108.3747, 37.3968) knots 0 0 0 0 1 1 1 1
  spline S2224 degree 3 poles (108.3747, 37.3968) (108.4214, 37.5708) (108.445, 37.7501) (108.445, 37.9301) knots 0 0 0 0 1 1 1 1
  spline S2225 degree 3 poles (12.4519, 76.2069) (12.916, 76.207) (13.361, 76.3914) (13.6891, 76.7195) knots 0 0 0 0 1 1 1 1
extrude "Extrude2" add sketch "test (1)" along normal blind 1 contours L0 L1 L2 L4 L5 L7 L8 L9 S12 L15 S13 L17 S15 L18 L20 L22 S27 L23 L24 L25 L27 L28 L31 L39 L573 L681 L682 L683 L684 S1558 L685 L686 L689 S1575 L690 L764 S1787 L768 L769 L770 L771 S1798 L781 L782 L783 L784 L786 L790 | L3 L6 S7 S10 L11 L12 L13 L14 L16 L21 S28 L26 L29 S918 S922 S927 S931 S946 S951 S957 S959 S960 S961 S962 S972 S980 S981 S998 S1003 S1023 S1024 L654 L655 L659 L661 L662 L663 S1522 L668 L669 L845 S2085 L847 S2086 S2088 L850 L859 L860 L861 S2092 L862 L864 L868 L871 L872 L874 L876 L881 L883 L884 L885 L888 | L30 L35 L183 L185 L192 S764 L249 L252 L253 S779 L254 L258 L264 L281 L473 L474 L475 L477 L478 L480 L485 L487 L488 L489 L490 L491 S1433 S1434 L492 L498 S1437 L501 L503 S1438 L504 L509 L723 L724 L725 S1709 L728 L729 L731 S1716 L733 L734 L802 L804 L805 L809 | L33 L36 L38 L40 L41 L44 L45 S79 L46 S83 L49 S85 L51 L52 L53 L54 L55 L56 L57 L58 S92 L60 S610 S612 S613 S620 S621 S628 S633 S634 S646 S1030 S1038 S1048 S1049 S1063 S1075 S1076 S1080 S1081 L647 L648 L649 L650 L651 L652 L653 L656 L658 S1518 L660 L664 L665 S1525 S1526 L666 L667 S1528 L670 L671 L672 L675 | S97 S98 S99 S105 S106 S108 S114 S118 S121 S141 S156 S161 S168 L75 S175 L78 S185 L80 S192 S194 L81 L82 L83 L84 L85 L86 S208 L88 L89 S838 S839 S848 S887 S892 S893 S904 S908 S914 L572 L579 L582 L583 L596 L600 S1471 S1473 L612 L613 L614 L616 L618 L619 S1484 S1485 L622 L627 S1488 S1489 S1490 S1493 L630 L632 L633 L634 L635 S1498 L637 L639 L641 L642 L644 L645 S1819 S1824 S1834 S1843 S1889 S1899 | S100 L74 L77 L87 S912 L574 L576 L577 L578 S1457 L580 L581 L584 L585 L586 S1459 L587 L588 L589 L590 S1460 L591 L592 L593 L594 L595 L597 L598 L599 S1464 L601 S1468 L605 L606 L610 L611 L615 L617 S1481 L623 L624 S1494 L638 L640 L643 S1510 L657 L673 L674 L676 | L92 L385 L386 L387 L388 L389 L390 L392 S1345 L394 L395 L396 L397 S1357 L398 S1364 L399 L400 L401 L402 L403 S1366 L404 L405 L524 L527 L528 L529 L530 L533 L534 L544 L545 L546 S1445 S1446 L548 S1447 L553 L554 L555 L556 S1452 L569 L575 L603 L933 L934 | L94 S351 L103 L105 L109 L126 L130 L131 S394 L135 L136 S397 L139 L140 L144 L151 L152 L153 L154 L156 S402 L159 L189 L190 L193 L194 L195 L196 L197 L198 S555 L200 L201 L203 S561 L205 L209 L210 S579 L211 L212 L213 S585 L217 L221 L338 L343 L356 L360 L361 | L95 L96 L97 L98 L100 S361 S364 L102 S370 L104 L106 L107 L108 L110 L111 L112 L113 L114 L115 L116 L117 S382 L199 L202 L204 L206 L207 S580 L214 L215 L216 L218 S586 L219 L823 L831 L832 L920 S2195 L923 L924 L925 L926 L927 L928 L929 L930 S2198 | L118 L119 L124 S386 L127 L128 S389 S390 L133 L134 L137 L138 L141 L142 L143 L145 L147 S400 L155 L157 L158 L160 L745 L746 L747 S1765 L750 L751 L752 L755 L756 S1780 L760 L761 L765 L766 L767 S1791 L773 L774 L775 S1797 L780 L785 L789 L826 L827 L828 L829 L830 | S383 S384 L120 L121 L122 L123 S385 L125 S387 L129 S388 S391 S392 S393 L132 S396 S398 L148 L149 L150 S399 S401 L161 L162 L163 L164 S403 L165 L166 S404 S405 S406 S407 S408 S409 S410 S412 S413 L167 L168 S414 S415 L169 S416 S420 L171 L172 L175 L744 S1746 L748 L749 L753 S1775 L757 L758 L759 L762 L763 L772 L776 L778 L779 L787 L788 L791 L792 L793 L794 S1820 S1840 L799 | S524 S558 S559 S568 S571 S597 S680 S684 S687 S1096 S1098 S1102 S1106 S1107 S1119 S1128 S1131 S1156 L421 L429 L433 L434 L435 L436 L439 L440 L441 S1423 L443 S1424 L447 L448 S1425 L450 L452 S1426 L455 L456 L465 L466 S2081 L849 L863 L865 S2095 L870 L875 S2097 L877 L878 L889 L890 L892 L893 L896 L897 L899 S2118 L903 L904 L910 L911 | S654 S666 S686 S692 S694 S698 S714 S718 S755 S1150 S1158 S1160 S1173 S1188 S1189 S1205 S1230 S1234 L422 L423 S1420 L425 L428 L431 L432 L437 S1422 L438 L445 L446 L453 L457 L458 L460 L461 S1428 L463 L464 L467 S1430 S2084 L846 L848 L851 L852 L853 L854 L855 L856 L857 L858 S2093 L866 L867 L869 S2096 L873 S2098 L880 L882 L886 L887 | L241 L242 L248 S1409 L414 L415 L416 L417 L419 L424 L426 L427 L430 S1421 L442 L444 L449 S1427 L459 L462 S1429 L602 L604 L607 L608 L691 L692 L693 L694 L695 L696 L697 L698 S1611 S1613 L699 L700 S1617 L702 L703 L704 L705 L706 L707 L708 S1627 L709 L710 | L321 L322 L323 L327 L331 L333 S1174 L337 L364 S1280 L366 L369 L370 L373 L374 L375 L376 S1310 L379 S1311 L380 L381 L384 S1443 L523 L525 L526 L535 L536 L537 L538 L539 L540 L541 L550 L552 L557 S1450 L565 L566 L568 S1453 L570 L571 S1454 L837 L838 L918 | L348 L349 L350 L351 L352 L353 L354 L355 S1247 S1259 L359 L362 L363 L365 S1289 L367 L368 L371 L372 L377 L378 L382 S1324 L520 L521 L522 L531 L532 L542 L543 S1444 L547 L549 L551 S1448 S1449 L558 L559 L560 S1451 L561 L562 L563 L564 L567 L720 L726 L922 | S1405 S1418 S1419 L451 L454 L468 L469 L470 S1431 L471 L472 S1432 L476 L479 L481 L482 L483 L484 L486 S1435 L493 L494 L495 L496 L497 L499 S1436 L500 L502 S1439 L505 L506 L507 S1440 S1441 L508 L510 L511 L512 L513 L514 S1442 L515 L516 L517 L518 L519 S1982 S1984 S1986 S1991 S1992 S1994 S2013 S2025 S2026 S2039 S2052 S2053 S2145 S2168 S2191 makes body 1 at (74.3628, 49.7788, 0) makes body 2 at (99.313, 24.9636, 0) makes body 3 at (107.8002, 78.0448, 0) makes body 4 at (49.1575, 67.3172, 0) makes body 5 at (34.6748, 55.7716, 0) makes body 6 at (93.2171, 80.6984, 0) makes body 7 at (118.3612, 23.1274, 0) makes body 8 at (70.0921, 69.3761, 0) makes body 9 at (50.0506, 50.3336, 0) makes body 10 at (88.3991, 49.3748, 0) makes body 11 at (107.2066, 61.0552, 0) makes body 12 at (52.6718, 81.917, 0) makes body 13 at (16.7432, 54.2027, 0) makes body 14 at (73.9108, 83.4908, 0) makes body 15 at (106.616, 44.0584, 0) makes body 16 at (88.693, 66.3793, 0) makes body 17 at (31.6758, 41.0513, 0)
extrude "Extrude1" add sketch "test (1)" along normal blind 4 separate body makes body 18
